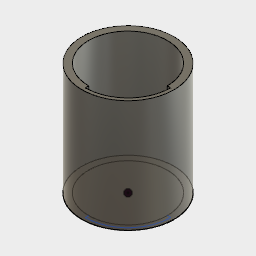
Gelatin_Mold_Outer v4 (Autodesk Fusion 360 design; units mm, degrees)
Autodesk Fusion 360 part; units mm, degrees
sketch "Sketch1" plane through (0, 0, 0) normal (0, 1, 0) x (1, 0, 0)
  circle A0 centre (0, 0) radius 41
  circle A1 centre (0, 0) radius 35
  line L0 (0.0406, -35) -> (0.0406, -38)
  line L1 (35, 0.0176) -> (38, 0.0176)
  arc A2 (0.0406, -38) -> (38, 0.0176) centre (0, 0) ccw
  dimension "d1" = 82
  dimension "d2" = 70
  measures "d1" diameter of A0
  measures "d2" diameter of A1
extrude "Extrude1" add sketch "Sketch1" along normal blind 100
extrude "Extrude2" add sketch "Sketch1" along normal blind 6 contours A1
extrude "Extrude3" add sketch "Sketch1" along normal blind 6 contours A1 L0 L1 A2
sketch "Sketch2" plane through (0, 6, 0) normal (0, 1, 0) x (-1, 0, 0)
  line L0 (-0.0406, 35) -> (-0.0406, 38)
  arc A0 (-0.0406, 38) -> (-38, -0.0176) centre (0, 0) ccw
  line L1 (-38, -0.0176) -> (-35, -0.0176)
  circle A1 centre (0, 0) radius 26
  arc A2 (-35, -0.0176) -> (-0.0406, 35) centre (0, 0) ccw
  dimension "d10" = 52
  measures "d10" diameter of A1
extrude "Extrude4" cut sketch "Sketch2" against normal blind 4 contours A1
